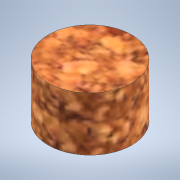
# Autodesk Inventor part: bulkhead
Saved by Autodesk Inventor 2021 (Build 250183000, 183)
## iProperties
Created: 2021-04-18
Part Number: bulkhead
Material: Concrete
Document SubType Name: Modeling
Designer: samlo
Density: 2.40731 g/cm^3
Appearance: Cork - Coarse
Author: samlo
Autodesk Inventor part; units mm, degrees
ref_plane "YZ Plane" through (0, 0, 0) normal (1, 0, 0) x (0, 1, 0)
ref_plane "XZ Plane" through (0, 0, 0) normal (0, 1, 0) x (-1, 0, 0)
ref_plane "XY Plane" through (0, 0, 0) normal (0, 0, 1) x (1, 0, 0)
sketch "Sketch1" plane through (0, 0, 0) normal (0, 0, 1) x (1, 0, 0)
  line L0 (0, 0) -> (15.5, 0)
  line L1 (15.5, 0) -> (15.5, 20)
  line L2 (15.5, 20) -> (0, 20)
  line L3 (0, 20) -> (0, 0)
  dimension "d0" = 20
  dimension "d1" = 15.5
  constraints: 8 end point, 2 parallel, 1 horizontal, 1 perpendicular
  measures "d0" distance of L2.end L0.start
  measures "d1" distance of L0.start L0.end
revolve "Revolution1" add sketch "Sketch1" angle 360 about axis through (0, 20, 0) along (0, -1, 0)
body "Solid1"
